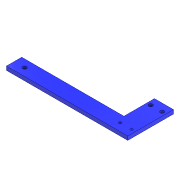
# Autodesk Inventor part: y_axis_extensor
Saved by Autodesk Inventor 2022 (Build 260153000, 153)
## iProperties
Created: 2021-09-30
Part Number: y_axis_extensor
Material: Generic
Document SubType Name: Modeling
Designer: nnico
Density: 1 g/cm^3
Appearance: Blue - Wall Paint - Glossy
Author: nnico
Autodesk Inventor part; units mm, degrees
ref_plane "YZ Plane" through (0, 0, 0) normal (1, 0, 0) x (0, 1, 0)
ref_plane "XZ Plane" through (0, 0, 0) normal (0, 1, 0) x (-1, 0, 0)
ref_plane "XY Plane" through (0, 0, 0) normal (0, 0, 1) x (1, 0, 0)
sketch "Sketch1" plane through (0, 0, 0) normal (0, 1, 0) x (-1, 0, 0)
  line L0 (12.5, -50) -> (-12.5, -50)
  line L1 (-12.5, -50) -> (-12.5, 10)
  line L2 (-12.5, 10) -> (12.5, 10)
  line L3 (12.5, 10) -> (12.5, -50)
  line L4 (12.5, 0) -> (-12.5, 0) construction
  line L5 (0, -50) -> (0, 10) construction
  circle A0 centre (7.5, 0) radius 1.6
  line L6 (12.5, 10) -> (146.5, 10)
  line L7 (146.5, 10) -> (146.5, -10)
  line L8 (146.5, -10) -> (12.5, -10)
  line L9 (12.5, -10) -> (12.5, 10)
  line L10 (146.5, 0) -> (12.5, 0) construction
  circle A1 centre (132.7538, 0) radius 2.5
  circle A2 centre (-7.5, 0) radius 1.6
  line L11 (12.5, -40) -> (-12.5, -40) construction
  circle A3 centre (7.5, -40) radius 2.5
  circle A4 centre (-7.5, -40) radius 2.5
  point P0 (0, 0)
  point P1 (0, 0)
  point P2 (12.5, -10)
  dimension "d0" = 3.2
  dimension "d1" = 15
  dimension "d3" = 10
  dimension "d4" = 60
  dimension "d5" = 25
  dimension "d6" = 134
  dimension "d7" = 20
  dimension "d8" = 5
  dimension "d9" = 10
  dimension "d10" = 5
  dimension "d11" = 15
  constraints: 24 end point, 7 point on line, 5 centre point, 4 midpoint, 4 parallel, 4 perpendicular, 2 horizontal, 2 symmetric about line, 1 coincident, 2 other
  measures "d0" diameter of A0
  measures "d1" diameter of A0.centre L5
  measures "d3" distance of L1.end L4.end
  measures "d4" distance of L0.end L1.end
  measures "d5" distance of L0.start L0.end
  measures "d6" distance of L7.end L8.end
  measures "d7" distance of L6.end L7.end
  measures "d8" diameter of A1
  measures "d9" distance of L0.start L11.start
  measures "d10" diameter of A3
  measures "d11" diameter of A3.centre L5
extrude "Extrusion1" add sketch "Sketch1" along normal blind 4
sketch "Sketch2" plane through (0, 0, 0) normal (0, -1, 0) x (1, 0, 0)
  line L0 (-146.5, 10) -> (12.5, 10) projected
  line L1 (-146.5, -10) -> (-146.5, 10) projected
  line L2 (-12.5, -10) -> (-146.5, -10) projected
  line L3 (-12.5, -50) -> (-12.5, -10) projected
  line L4 (12.5, -50) -> (-12.5, -50) projected
  line L5 (12.5, 10) -> (12.5, -50) projected
  circle A0 centre (-7.5, 0) radius 1.6 projected
  circle A1 centre (7.5, 0) radius 1.6 projected
  circle A2 centre (-7.5, -40) radius 2.5 projected
  circle A3 centre (7.5, -40) radius 2.5 projected
  circle A4 centre (-132.7538, 0) radius 2.5 projected
extrude "Extrusion2" add sketch "Sketch2" along normal blind 1 contours L0 L5 L4 L3 L2 L1 | A2 | A3 | A4
body "Solid1"
